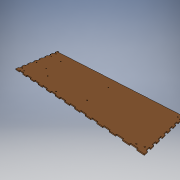
# Autodesk Inventor part: tavolaBase
Saved by Autodesk Inventor 2018.3 (Build 223284000, 284)
## iProperties
Created: 2019-03-04
Part Number: tavolaBase
Material: Generico
Document SubType Name: Modeling
Designer: AlfyPc
Density: 1 g/cm^3
Appearance: Frassino bianco - Giava
Author: AlfyPc
Autodesk Inventor part; units mm, degrees
ref_plane "YZ Plane" through (0, 0, 0) normal (1, 0, 0) x (0, 1, 0)
ref_plane "XZ Plane" through (0, 0, 0) normal (0, 1, 0) x (-1, 0, 0)
ref_plane "XY Plane" through (0, 0, 0) normal (0, 0, 1) x (1, 0, 0)
sketch "Schizzo1" plane through (0, 0, 0) normal (0, 0, 1) x (1, 0, 0)
  line L0 (233.5, -78.5) -> (-233.5, -78.5)
  line L1 (-233.5, -78.5) -> (-233.5, 78.5)
  line L2 (-233.5, 78.5) -> (233.5, 78.5)
  line L3 (233.5, 78.5) -> (233.5, -78.5)
  line L4 (233.5, -78.5) -> (-233.5, 78.5) construction
  line L5 (-233.5, -78.5) -> (233.5, 78.5) construction
  point P0 (0, 0)
  dimension "d0" = 467
  dimension "d1" = 157
  constraints: 12 end point, 2 midpoint, 2 parallel, 1 horizontal, 1 perpendicular
  measures "d0" distance of L0.start L0.end
  measures "d1" distance of L0.end L1.end
extrude "Estrusione1" add sketch "Schizzo1" against normal blind 4
sketch "Schizzo3" plane through (0, 0, 0) normal (0, 0, 1) x (1, 0, 0)
  line L0 (233.5, -78.5) -> (-233.5, -78.5) projected
  line L1 (233.5, 78.5) -> (233.5, -78.5) projected
  line L2 (-233.5, 78.5) -> (233.5, 78.5) projected
  line L3 (-233.5, -78.5) -> (-233.5, 78.5) projected
  line L4 (-237.5, -82.5) -> (237.5, -82.5) construction
  line L5 (237.5, -82.5) -> (237.5, 82.5) construction
  line L6 (237.5, 82.5) -> (-237.5, 82.5) construction
  line L7 (-237.5, 82.5) -> (-237.5, -82.5) construction
  line L8 (237.5, -82.5) -> (218.5, -82.5)
  line L9 (218.5, -82.5) -> (218.5, -78.5)
  line L10 (218.5, -78.5) -> (237.5, -78.5)
  line L11 (237.5, -78.5) -> (237.5, -82.5)
  line L12 (237.5, 82.5) -> (218.5, 82.5)
  line L13 (218.5, 82.5) -> (218.5, 78.5)
  line L14 (218.5, 78.5) -> (237.5, 78.5)
  line L15 (237.5, 78.5) -> (237.5, 82.5)
  line L16 (237.5, -82.5) -> (233.5, -82.5)
  line L17 (233.5, -82.5) -> (233.5, -71.5)
  line L18 (233.5, -71.5) -> (237.5, -71.5)
  line L19 (237.5, -71.5) -> (237.5, -82.5)
  line L20 (-237.5, -82.5) -> (-233.5, -82.5)
  line L21 (-233.5, -82.5) -> (-233.5, -71.5)
  line L22 (-233.5, -71.5) -> (-237.5, -71.5)
  line L23 (-237.5, -71.5) -> (-237.5, -82.5)
  line L24 (218.5, -78.5) -> (218.5, -82.5)
  line L25 (218.5, -82.5) -> (214.5, -82.5)
  line L26 (199.5, -82.5) -> (199.5, -78.5)
  line L27 (199.5, -78.5) -> (218.5, -78.5)
  line L28 (218.5, -82.5) -> (199.5, -82.5)
  line L29 (199.5, 82.5) -> (199.5, 78.5)
  line L30 (199.5, 78.5) -> (218.5, 78.5)
  line L31 (218.5, 78.5) -> (218.5, 82.5)
  line L32 (218.5, 82.5) -> (199.5, 82.5)
  line L33 (199.5, -78.5) -> (199.5, -82.5)
  line L34 (199.5, -82.5) -> (195.5, -82.5)
  line L35 (180.5, -82.5) -> (180.5, -78.5)
  line L36 (180.5, -78.5) -> (199.5, -78.5)
  line L37 (199.5, -82.5) -> (180.5, -82.5)
  line L38 (180.5, 82.5) -> (180.5, 78.5)
  line L39 (180.5, 78.5) -> (199.5, 78.5)
  line L40 (199.5, 78.5) -> (199.5, 82.5)
  line L41 (199.5, 82.5) -> (180.5, 82.5)
  line L42 (180.5, -78.5) -> (180.5, -82.5)
  line L43 (180.5, -82.5) -> (176.5, -82.5)
  line L44 (161.5, -82.5) -> (161.5, -78.5)
  line L45 (161.5, -78.5) -> (180.5, -78.5)
  line L46 (180.5, -82.5) -> (161.5, -82.5)
  line L47 (161.5, 82.5) -> (161.5, 78.5)
  line L48 (161.5, 78.5) -> (180.5, 78.5)
  line L49 (180.5, 78.5) -> (180.5, 82.5)
  line L50 (180.5, 82.5) -> (161.5, 82.5)
  line L51 (161.5, -78.5) -> (161.5, -82.5)
  line L52 (161.5, -82.5) -> (157.5, -82.5)
  line L53 (142.5, -82.5) -> (142.5, -78.5)
  line L54 (142.5, -78.5) -> (161.5, -78.5)
  line L55 (161.5, -82.5) -> (142.5, -82.5)
  line L56 (142.5, 82.5) -> (142.5, 78.5)
  line L57 (142.5, 78.5) -> (161.5, 78.5)
  line L58 (161.5, 78.5) -> (161.5, 82.5)
  line L59 (161.5, 82.5) -> (142.5, 82.5)
  line L60 (142.5, -78.5) -> (142.5, -82.5)
  line L61 (142.5, -82.5) -> (138.5, -82.5)
  line L62 (123.5, -82.5) -> (123.5, -78.5)
  line L63 (123.5, -78.5) -> (142.5, -78.5)
  line L64 (142.5, -82.5) -> (123.5, -82.5)
  line L65 (123.5, 82.5) -> (123.5, 78.5)
  line L66 (123.5, 78.5) -> (142.5, 78.5)
  line L67 (142.5, 78.5) -> (142.5, 82.5)
  line L68 (142.5, 82.5) -> (123.5, 82.5)
  line L69 (123.5, -78.5) -> (123.5, -82.5)
  line L70 (123.5, -82.5) -> (119.5, -82.5)
  line L71 (104.5, -82.5) -> (104.5, -78.5)
  line L72 (104.5, -78.5) -> (123.5, -78.5)
  line L73 (123.5, -82.5) -> (104.5, -82.5)
  line L74 (104.5, 82.5) -> (104.5, 78.5)
  line L75 (104.5, 78.5) -> (123.5, 78.5)
  line L76 (123.5, 78.5) -> (123.5, 82.5)
  line L77 (123.5, 82.5) -> (104.5, 82.5)
  line L78 (104.5, -78.5) -> (104.5, -82.5)
  line L79 (104.5, -82.5) -> (100.5, -82.5)
  line L80 (85.5, -82.5) -> (85.5, -78.5)
  line L81 (85.5, -78.5) -> (104.5, -78.5)
  line L82 (104.5, -82.5) -> (85.5, -82.5)
  line L83 (85.5, 82.5) -> (85.5, 78.5)
  line L84 (85.5, 78.5) -> (104.5, 78.5)
  line L85 (104.5, 78.5) -> (104.5, 82.5)
  line L86 (104.5, 82.5) -> (85.5, 82.5)
  line L87 (85.5, -78.5) -> (85.5, -82.5)
  line L88 (85.5, -82.5) -> (81.5, -82.5)
  line L89 (66.5, -82.5) -> (66.5, -78.5)
  line L90 (66.5, -78.5) -> (85.5, -78.5)
  line L91 (85.5, -82.5) -> (66.5, -82.5)
  line L92 (66.5, 82.5) -> (66.5, 78.5)
  line L93 (66.5, 78.5) -> (85.5, 78.5)
  line L94 (85.5, 78.5) -> (85.5, 82.5)
  line L95 (85.5, 82.5) -> (66.5, 82.5)
  line L96 (66.5, -78.5) -> (66.5, -82.5)
  line L97 (66.5, -82.5) -> (62.5, -82.5)
  line L98 (47.5, -82.5) -> (47.5, -78.5)
  line L99 (47.5, -78.5) -> (66.5, -78.5)
  line L100 (66.5, -82.5) -> (47.5, -82.5)
  line L101 (47.5, 82.5) -> (47.5, 78.5)
  line L102 (47.5, 78.5) -> (66.5, 78.5)
  line L103 (66.5, 78.5) -> (66.5, 82.5)
  line L104 (66.5, 82.5) -> (47.5, 82.5)
  line L105 (47.5, -78.5) -> (47.5, -82.5)
  line L106 (47.5, -82.5) -> (43.5, -82.5)
  line L107 (28.5, -82.5) -> (28.5, -78.5)
  line L108 (28.5, -78.5) -> (47.5, -78.5)
  line L109 (47.5, -82.5) -> (28.5, -82.5)
  line L110 (28.5, 82.5) -> (28.5, 78.5)
  line L111 (28.5, 78.5) -> (47.5, 78.5)
  line L112 (47.5, 78.5) -> (47.5, 82.5)
  line L113 (47.5, 82.5) -> (28.5, 82.5)
  line L114 (28.5, -78.5) -> (28.5, -82.5)
  line L115 (28.5, -82.5) -> (24.5, -82.5)
  line L116 (9.5, -82.5) -> (9.5, -78.5)
  line L117 (9.5, -78.5) -> (28.5, -78.5)
  line L118 (28.5, -82.5) -> (9.5, -82.5)
  line L119 (9.5, 82.5) -> (9.5, 78.5)
  line L120 (9.5, 78.5) -> (28.5, 78.5)
  line L121 (28.5, 78.5) -> (28.5, 82.5)
  line L122 (28.5, 82.5) -> (9.5, 82.5)
  line L123 (9.5, -78.5) -> (9.5, -82.5)
  line L124 (9.5, -82.5) -> (5.5, -82.5)
  line L125 (-9.5, -82.5) -> (-9.5, -78.5)
  line L126 (-9.5, -78.5) -> (9.5, -78.5)
  line L127 (9.5, -82.5) -> (-9.5, -82.5)
  line L128 (-9.5, 82.5) -> (-9.5, 78.5)
  line L129 (-9.5, 78.5) -> (9.5, 78.5)
  line L130 (9.5, 78.5) -> (9.5, 82.5)
  line L131 (9.5, 82.5) -> (-9.5, 82.5)
  line L132 (-9.5, -78.5) -> (-9.5, -82.5)
  line L133 (-9.5, -82.5) -> (-13.5, -82.5)
  line L134 (-28.5, -82.5) -> (-28.5, -78.5)
  line L135 (-28.5, -78.5) -> (-9.5, -78.5)
  line L136 (-9.5, -82.5) -> (-28.5, -82.5)
  line L137 (-28.5, 82.5) -> (-28.5, 78.5)
  line L138 (-28.5, 78.5) -> (-9.5, 78.5)
  line L139 (-9.5, 78.5) -> (-9.5, 82.5)
  line L140 (-9.5, 82.5) -> (-28.5, 82.5)
  line L141 (-28.5, -78.5) -> (-28.5, -82.5)
  line L142 (-28.5, -82.5) -> (-32.5, -82.5)
  line L143 (-47.5, -82.5) -> (-47.5, -78.5)
  line L144 (-47.5, -78.5) -> (-28.5, -78.5)
  line L145 (-28.5, -82.5) -> (-47.5, -82.5)
  line L146 (-47.5, 82.5) -> (-47.5, 78.5)
  line L147 (-47.5, 78.5) -> (-28.5, 78.5)
  line L148 (-28.5, 78.5) -> (-28.5, 82.5)
  line L149 (-28.5, 82.5) -> (-47.5, 82.5)
  line L150 (-47.5, -78.5) -> (-47.5, -82.5)
  line L151 (-47.5, -82.5) -> (-51.5, -82.5)
  line L152 (-66.5, -82.5) -> (-66.5, -78.5)
  line L153 (-66.5, -78.5) -> (-47.5, -78.5)
  line L154 (-47.5, -82.5) -> (-66.5, -82.5)
  line L155 (-66.5, 82.5) -> (-66.5, 78.5)
  line L156 (-66.5, 78.5) -> (-47.5, 78.5)
  line L157 (-47.5, 78.5) -> (-47.5, 82.5)
  line L158 (-47.5, 82.5) -> (-66.5, 82.5)
  line L159 (-66.5, -78.5) -> (-66.5, -82.5)
  line L160 (-66.5, -82.5) -> (-70.5, -82.5)
  line L161 (-85.5, -82.5) -> (-85.5, -78.5)
  line L162 (-85.5, -78.5) -> (-66.5, -78.5)
  line L163 (-66.5, -82.5) -> (-85.5, -82.5)
  line L164 (-85.5, 82.5) -> (-85.5, 78.5)
  line L165 (-85.5, 78.5) -> (-66.5, 78.5)
  line L166 (-66.5, 78.5) -> (-66.5, 82.5)
  line L167 (-66.5, 82.5) -> (-85.5, 82.5)
  line L168 (-85.5, -78.5) -> (-85.5, -82.5)
  line L169 (-85.5, -82.5) -> (-89.5, -82.5)
  line L170 (-104.5, -82.5) -> (-104.5, -78.5)
  line L171 (-104.5, -78.5) -> (-85.5, -78.5)
  line L172 (-85.5, -82.5) -> (-104.5, -82.5)
  line L173 (-104.5, 82.5) -> (-104.5, 78.5)
  line L174 (-104.5, 78.5) -> (-85.5, 78.5)
  line L175 (-85.5, 78.5) -> (-85.5, 82.5)
  line L176 (-85.5, 82.5) -> (-104.5, 82.5)
  line L177 (-104.5, -78.5) -> (-104.5, -82.5)
  line L178 (-104.5, -82.5) -> (-108.5, -82.5)
  line L179 (-123.5, -82.5) -> (-123.5, -78.5)
  line L180 (-123.5, -78.5) -> (-104.5, -78.5)
  line L181 (-104.5, -82.5) -> (-123.5, -82.5)
  line L182 (-123.5, 82.5) -> (-123.5, 78.5)
  line L183 (-123.5, 78.5) -> (-104.5, 78.5)
  line L184 (-104.5, 78.5) -> (-104.5, 82.5)
  line L185 (-104.5, 82.5) -> (-123.5, 82.5)
  line L186 (-123.5, -78.5) -> (-123.5, -82.5)
  line L187 (-123.5, -82.5) -> (-127.5, -82.5)
  line L188 (-142.5, -82.5) -> (-142.5, -78.5)
  line L189 (-142.5, -78.5) -> (-123.5, -78.5)
  line L190 (-123.5, -82.5) -> (-142.5, -82.5)
  line L191 (-142.5, 82.5) -> (-142.5, 78.5)
  line L192 (-142.5, 78.5) -> (-123.5, 78.5)
  line L193 (-123.5, 78.5) -> (-123.5, 82.5)
  line L194 (-123.5, 82.5) -> (-142.5, 82.5)
  line L195 (-142.5, -78.5) -> (-142.5, -82.5)
  line L196 (-142.5, -82.5) -> (-146.5, -82.5)
  line L197 (-161.5, -82.5) -> (-161.5, -78.5)
  line L198 (-161.5, -78.5) -> (-142.5, -78.5)
  line L199 (-142.5, -82.5) -> (-161.5, -82.5)
  line L200 (-161.5, 82.5) -> (-161.5, 78.5)
  line L201 (-161.5, 78.5) -> (-142.5, 78.5)
  line L202 (-142.5, 78.5) -> (-142.5, 82.5)
  line L203 (-142.5, 82.5) -> (-161.5, 82.5)
  line L204 (-161.5, -78.5) -> (-161.5, -82.5)
  line L205 (-161.5, -82.5) -> (-165.5, -82.5)
  line L206 (-180.5, -82.5) -> (-180.5, -78.5)
  line L207 (-180.5, -78.5) -> (-161.5, -78.5)
  line L208 (-161.5, -82.5) -> (-180.5, -82.5)
  line L209 (-180.5, 82.5) -> (-180.5, 78.5)
  line L210 (-180.5, 78.5) -> (-161.5, 78.5)
  line L211 (-161.5, 78.5) -> (-161.5, 82.5)
  line L212 (-161.5, 82.5) -> (-180.5, 82.5)
  line L213 (-180.5, -78.5) -> (-180.5, -82.5)
  line L214 (-180.5, -82.5) -> (-184.5, -82.5)
  line L215 (-199.5, -82.5) -> (-199.5, -78.5)
  line L216 (-199.5, -78.5) -> (-180.5, -78.5)
  line L217 (-180.5, -82.5) -> (-199.5, -82.5)
  line L218 (-199.5, 82.5) -> (-199.5, 78.5)
  line L219 (-199.5, 78.5) -> (-180.5, 78.5)
  line L220 (-180.5, 78.5) -> (-180.5, 82.5)
  line L221 (-180.5, 82.5) -> (-199.5, 82.5)
  line L222 (-199.5, -78.5) -> (-199.5, -82.5)
  line L223 (-199.5, -82.5) -> (-203.5, -82.5)
  line L224 (-218.5, -82.5) -> (-218.5, -78.5)
  line L225 (-218.5, -78.5) -> (-199.5, -78.5)
  line L226 (-199.5, -82.5) -> (-218.5, -82.5)
  line L227 (-218.5, 82.5) -> (-218.5, 78.5)
  line L228 (-218.5, 78.5) -> (-199.5, 78.5)
  line L229 (-199.5, 78.5) -> (-199.5, 82.5)
  line L230 (-199.5, 82.5) -> (-218.5, 82.5)
  line L231 (-218.5, -78.5) -> (-218.5, -82.5)
  line L232 (-218.5, -82.5) -> (-222.5, -82.5)
  line L233 (-237.5, -82.5) -> (-237.5, -78.5)
  line L234 (-237.5, -78.5) -> (-218.5, -78.5)
  line L235 (-218.5, -82.5) -> (-237.5, -82.5)
  line L236 (-237.5, 82.5) -> (-237.5, 78.5)
  line L237 (-237.5, 78.5) -> (-218.5, 78.5)
  line L238 (-218.5, 78.5) -> (-218.5, 82.5)
  line L239 (-218.5, 82.5) -> (-237.5, 82.5)
  line L240 (237.5, -67.5) -> (237.5, -71.5)
  line L241 (237.5, -71.5) -> (233.5, -71.5)
  line L242 (233.5, -60.5) -> (237.5, -60.5)
  line L243 (237.5, -60.5) -> (237.5, -71.5)
  line L244 (233.5, -71.5) -> (233.5, -60.5)
  line L245 (-237.5, -71.5) -> (-233.5, -71.5)
  line L246 (-233.5, -71.5) -> (-233.5, -60.5)
  line L247 (-233.5, -60.5) -> (-237.5, -60.5)
  line L248 (-237.5, -60.5) -> (-237.5, -71.5)
  line L249 (-237.5, -71.5) -> (-237.5, -67.5)
  line L250 (237.5, -56.5) -> (237.5, -60.5)
  line L251 (237.5, -60.5) -> (233.5, -60.5)
  line L252 (233.5, -49.5) -> (237.5, -49.5)
  line L253 (237.5, -49.5) -> (237.5, -60.5)
  line L254 (233.5, -60.5) -> (233.5, -49.5)
  line L255 (-237.5, -60.5) -> (-233.5, -60.5)
  line L256 (-233.5, -60.5) -> (-233.5, -49.5)
  line L257 (-233.5, -49.5) -> (-237.5, -49.5)
  line L258 (-237.5, -49.5) -> (-237.5, -60.5)
  line L259 (-237.5, -60.5) -> (-237.5, -56.5)
  line L260 (237.5, -45.5) -> (237.5, -49.5)
  line L261 (237.5, -49.5) -> (233.5, -49.5)
  line L262 (233.5, -38.5) -> (237.5, -38.5)
  line L263 (237.5, -38.5) -> (237.5, -49.5)
  line L264 (233.5, -49.5) -> (233.5, -38.5)
  line L265 (-237.5, -49.5) -> (-233.5, -49.5)
  line L266 (-233.5, -49.5) -> (-233.5, -38.5)
  line L267 (-233.5, -38.5) -> (-237.5, -38.5)
  line L268 (-237.5, -38.5) -> (-237.5, -49.5)
  line L269 (-237.5, -49.5) -> (-237.5, -45.5)
  line L270 (237.5, -34.5) -> (237.5, -38.5)
  line L271 (237.5, -38.5) -> (233.5, -38.5)
  line L272 (233.5, -27.5) -> (237.5, -27.5)
  line L273 (237.5, -27.5) -> (237.5, -38.5)
  line L274 (233.5, -38.5) -> (233.5, -27.5)
  line L275 (-237.5, -38.5) -> (-233.5, -38.5)
  line L276 (-233.5, -38.5) -> (-233.5, -27.5)
  line L277 (-233.5, -27.5) -> (-237.5, -27.5)
  line L278 (-237.5, -27.5) -> (-237.5, -38.5)
  line L279 (-237.5, -38.5) -> (-237.5, -34.5)
  line L280 (237.5, -23.5) -> (237.5, -27.5)
  line L281 (237.5, -27.5) -> (233.5, -27.5)
  line L282 (233.5, -16.5) -> (237.5, -16.5)
  line L283 (237.5, -16.5) -> (237.5, -27.5)
  line L284 (233.5, -27.5) -> (233.5, -16.5)
  line L285 (-237.5, -27.5) -> (-233.5, -27.5)
  line L286 (-233.5, -27.5) -> (-233.5, -16.5)
  line L287 (-233.5, -16.5) -> (-237.5, -16.5)
  line L288 (-237.5, -16.5) -> (-237.5, -27.5)
  line L289 (-237.5, -27.5) -> (-237.5, -23.5)
  line L290 (237.5, -12.5) -> (237.5, -16.5)
  line L291 (237.5, -16.5) -> (233.5, -16.5)
  line L292 (233.5, -5.5) -> (237.5, -5.5)
  line L293 (237.5, -5.5) -> (237.5, -16.5)
  line L294 (233.5, -16.5) -> (233.5, -5.5)
  line L295 (-237.5, -16.5) -> (-233.5, -16.5)
  line L296 (-233.5, -16.5) -> (-233.5, -5.5)
  line L297 (-233.5, -5.5) -> (-237.5, -5.5)
  line L298 (-237.5, -5.5) -> (-237.5, -16.5)
  line L299 (-237.5, -16.5) -> (-237.5, -12.5)
  line L300 (237.5, -1.5) -> (237.5, -5.5)
  line L301 (237.5, -5.5) -> (233.5, -5.5)
  line L302 (233.5, 5.5) -> (237.5, 5.5)
  line L303 (237.5, 5.5) -> (237.5, -5.5)
  line L304 (233.5, -5.5) -> (233.5, 5.5)
  line L305 (-237.5, -5.5) -> (-233.5, -5.5)
  line L306 (-233.5, -5.5) -> (-233.5, 5.5)
  line L307 (-233.5, 5.5) -> (-237.5, 5.5)
  line L308 (-237.5, 5.5) -> (-237.5, -5.5)
  line L309 (-237.5, -5.5) -> (-237.5, -1.5)
  line L310 (237.5, 9.5) -> (237.5, 5.5)
  line L311 (237.5, 5.5) -> (233.5, 5.5)
  line L312 (233.5, 16.5) -> (237.5, 16.5)
  line L313 (237.5, 16.5) -> (237.5, 5.5)
  line L314 (233.5, 5.5) -> (233.5, 16.5)
  line L315 (-237.5, 5.5) -> (-233.5, 5.5)
  line L316 (-233.5, 5.5) -> (-233.5, 16.5)
  line L317 (-233.5, 16.5) -> (-237.5, 16.5)
  line L318 (-237.5, 16.5) -> (-237.5, 5.5)
  line L319 (-237.5, 5.5) -> (-237.5, 9.5)
  line L320 (237.5, 20.5) -> (237.5, 16.5)
  line L321 (237.5, 16.5) -> (233.5, 16.5)
  line L322 (233.5, 27.5) -> (237.5, 27.5)
  line L323 (237.5, 27.5) -> (237.5, 16.5)
  line L324 (233.5, 16.5) -> (233.5, 27.5)
  line L325 (-237.5, 16.5) -> (-233.5, 16.5)
  line L326 (-233.5, 16.5) -> (-233.5, 27.5)
  line L327 (-233.5, 27.5) -> (-237.5, 27.5)
  line L328 (-237.5, 27.5) -> (-237.5, 16.5)
  line L329 (-237.5, 16.5) -> (-237.5, 20.5)
  line L330 (237.5, 31.5) -> (237.5, 27.5)
  line L331 (237.5, 27.5) -> (233.5, 27.5)
  line L332 (233.5, 38.5) -> (237.5, 38.5)
  line L333 (237.5, 38.5) -> (237.5, 27.5)
  line L334 (233.5, 27.5) -> (233.5, 38.5)
  line L335 (-237.5, 27.5) -> (-233.5, 27.5)
  line L336 (-233.5, 27.5) -> (-233.5, 38.5)
  line L337 (-233.5, 38.5) -> (-237.5, 38.5)
  line L338 (-237.5, 38.5) -> (-237.5, 27.5)
  line L339 (-237.5, 27.5) -> (-237.5, 31.5)
  line L340 (237.5, 42.5) -> (237.5, 38.5)
  line L341 (237.5, 38.5) -> (233.5, 38.5)
  line L342 (233.5, 49.5) -> (237.5, 49.5)
  line L343 (237.5, 49.5) -> (237.5, 38.5)
  line L344 (233.5, 38.5) -> (233.5, 49.5)
  line L345 (-237.5, 38.5) -> (-233.5, 38.5)
  line L346 (-233.5, 38.5) -> (-233.5, 49.5)
  line L347 (-233.5, 49.5) -> (-237.5, 49.5)
  line L348 (-237.5, 49.5) -> (-237.5, 38.5)
  line L349 (-237.5, 38.5) -> (-237.5, 42.5)
  line L350 (237.5, 53.5) -> (237.5, 49.5)
  line L351 (237.5, 49.5) -> (233.5, 49.5)
  line L352 (233.5, 60.5) -> (237.5, 60.5)
  line L353 (237.5, 60.5) -> (237.5, 49.5)
  line L354 (233.5, 49.5) -> (233.5, 60.5)
  line L355 (-237.5, 49.5) -> (-233.5, 49.5)
  line L356 (-233.5, 49.5) -> (-233.5, 60.5)
  line L357 (-233.5, 60.5) -> (-237.5, 60.5)
  line L358 (-237.5, 60.5) -> (-237.5, 49.5)
  line L359 (-237.5, 49.5) -> (-237.5, 53.5)
  line L360 (237.5, 64.5) -> (237.5, 60.5)
  line L361 (237.5, 60.5) -> (233.5, 60.5)
  line L362 (233.5, 71.5) -> (237.5, 71.5)
  line L363 (237.5, 71.5) -> (237.5, 60.5)
  line L364 (233.5, 60.5) -> (233.5, 71.5)
  line L365 (-237.5, 60.5) -> (-233.5, 60.5)
  line L366 (-233.5, 60.5) -> (-233.5, 71.5)
  line L367 (-233.5, 71.5) -> (-237.5, 71.5)
  line L368 (-237.5, 71.5) -> (-237.5, 60.5)
  line L369 (-237.5, 60.5) -> (-237.5, 64.5)
  line L370 (237.5, 75.5) -> (237.5, 71.5)
  line L371 (237.5, 71.5) -> (233.5, 71.5)
  line L372 (233.5, 82.5) -> (237.5, 82.5)
  line L373 (237.5, 82.5) -> (237.5, 71.5)
  line L374 (233.5, 71.5) -> (233.5, 82.5)
  line L375 (-237.5, 71.5) -> (-233.5, 71.5)
  line L376 (-233.5, 71.5) -> (-233.5, 82.5)
  line L377 (-233.5, 82.5) -> (-237.5, 82.5)
  line L378 (-237.5, 82.5) -> (-237.5, 71.5)
  line L379 (-237.5, 71.5) -> (-237.5, 75.5)
  point P0 (0, 0)
  point P1 (214.5, -78.5)
  point P2 (214.5, 78.5)
  point P3 (195.5, -78.5)
  point P4 (195.5, 78.5)
  point P5 (176.5, -78.5)
  point P6 (176.5, 78.5)
  point P7 (157.5, -78.5)
  point P8 (157.5, 78.5)
  point P9 (138.5, -78.5)
  point P10 (138.5, 78.5)
  point P11 (119.5, -78.5)
  point P12 (119.5, 78.5)
  point P13 (100.5, -78.5)
  point P14 (100.5, 78.5)
  point P15 (81.5, -78.5)
  point P16 (81.5, 78.5)
  point P17 (62.5, -78.5)
  point P18 (62.5, 78.5)
  point P19 (43.5, -78.5)
  point P20 (43.5, 78.5)
  point P21 (24.5, -78.5)
  point P22 (24.5, 78.5)
  point P23 (5.5, -78.5)
  point P24 (5.5, 78.5)
  point P25 (-13.5, -78.5)
  point P26 (-13.5, 78.5)
  point P27 (-32.5, -78.5)
  point P28 (-32.5, 78.5)
  point P29 (-51.5, -78.5)
  point P30 (-51.5, 78.5)
  point P31 (-70.5, -78.5)
  point P32 (-70.5, 78.5)
  point P33 (-89.5, -78.5)
  point P34 (-89.5, 78.5)
  point P35 (-108.5, -78.5)
  point P36 (-108.5, 78.5)
  point P37 (-127.5, -78.5)
  point P38 (-127.5, 78.5)
  point P39 (-146.5, -78.5)
  point P40 (-146.5, 78.5)
  point P41 (-165.5, -78.5)
  point P42 (-165.5, 78.5)
  point P43 (-184.5, -78.5)
  point P44 (-184.5, 78.5)
  point P45 (-203.5, -78.5)
  point P46 (-203.5, 78.5)
  point P47 (-222.5, -78.5)
  point P48 (-222.5, 78.5)
  point P49 (233.5, -67.5)
  point P50 (-233.5, -67.5)
  point P51 (233.5, -56.5)
  point P52 (-233.5, -56.5)
  point P53 (233.5, -45.5)
  point P54 (-233.5, -45.5)
  point P55 (233.5, -34.5)
  point P56 (-233.5, -34.5)
  point P57 (233.5, -23.5)
  point P58 (-233.5, -23.5)
  point P59 (233.5, -12.5)
  point P60 (-233.5, -12.5)
  point P61 (233.5, -1.5)
  point P62 (-233.5, -1.5)
  point P63 (233.5, 9.5)
  point P64 (-233.5, 9.5)
  point P65 (233.5, 20.5)
  point P66 (-233.5, 20.5)
  point P67 (233.5, 31.5)
  point P68 (-233.5, 31.5)
  point P69 (233.5, 42.5)
  point P70 (-233.5, 42.5)
  point P71 (233.5, 53.5)
  point P72 (-233.5, 53.5)
  point P73 (233.5, 64.5)
  point P74 (-233.5, 64.5)
  point P75 (233.5, 75.5)
  point P76 (-233.5, 75.5)
  dimension "d28" = 4
  dimension "d29" = 475
  dimension "d30" = 165
  dimension "d31" = 19
  dimension "d32" = 4
  dimension "d33" = 19
  dimension "d34" = 4
  dimension "d35" = 4
  dimension "d36" = 11
  dimension "d37" = 4
  dimension "d38" = 11
  dimension "d41" = 19
  dimension "d48" = 11
  constraints: 752 end point, 8 parallel, 5 horizontal, 4 perpendicular, 1 vertical, 805 other
  measures "d28" distance between parallel lines of L0 L4
  measures "d29" distance of L4.start L4.end
  measures "d30" distance of L4.end L5.end
  measures "d31" distance of L9.end L10.end
  measures "d32" distance of L8.end L9.end
  measures "d33" distance of L14.end L13.end
  measures "d34" distance of L13.end L12.end
  measures "d35" distance of L17.end L18.end
  measures "d36" distance of L16.end L17.end
  measures "d37" distance of L22.end L21.end
  measures "d38" distance of L21.end L20.end
  measures "d41" distance of L10.end L24.start
  measures "d48" distance of L0.start point (233.5, -67.5)
extrude "Estrusione2" add sketch "Schizzo3" against normal up to surface (4 mm away) contours L17 L8 L9 L0 | L1 L18 L19 L10 | L10 L11 L8 L17 | L26 L34 L37 L35 L0 | L1 L252 L253 L250 L242 | L44 L52 L55 L53 L0 | L1 L272 L273 L270 L262 | L62 L70 L73 L71 L0 | L1 L292 L293 L290 L282 | L80 L88 L91 L89 L0 | L1 L312 L313 L310 L302 | L98 L106 L109 L107 L0 | L1 L332 L333 L330 L322 | L116 L124 L127 L125 L0 | L1 L352 L353 L350 L342 | L134 L142 L145 L143 L0 | L1 L14 L373 L370 L362 | L374 L12 L15 L14 | L152 L160 L163 L161 L0 | L170 L178 L181 L179 L0 | L188 L196 L199 L197 L0 | L206 L214 L217 L215 L0 | L224 L232 L235 L21 L0 | L234 L23 L22 L3 | L21 L20 L23 L234 | L247 L258 L257 L3 | L267 L278 L277 L3 | L287 L298 L297 L3 | L307 L318 L317 L3 | L327 L338 L337 L3 | L347 L358 L357 L3 | L367 L378 L237 L3 | L237 L236 L239 L376
sketch "Schizzo4" plane through (0, 0, 0) normal (0, 0, 1) x (1, 0, 0)
  circle A0 centre (29.075, -39.395) radius 1.5
  circle A1 centre (29.075, 41.885) radius 1.5
  circle A2 centre (-135.39, -38.76) radius 1.5
  circle A3 centre (-173.97, 42.5) radius 1.375
  circle A4 centre (-222.97, 42.5) radius 1.375
  circle A5 centre (-173.97, -15.5) radius 1.375
  circle A6 centre (-222.97, -15.5) radius 1.375
  point P0 (0, 0)
extrude "Estrusione3" cut sketch "Schizzo4" against normal blind 10
sketch "Schizzo5" plane through (0, 0, 0) normal (0, 0, 1) x (1, 0, 0)
  circle A0 centre (29.075, 41.885) radius 1.5 projected
  circle A1 centre (-222.97, -15.5) radius 1.375 projected
  circle A2 centre (-222.97, 42.5) radius 1.375 projected
  circle A3 centre (-173.97, 42.5) radius 1.375 projected
  circle A4 centre (-173.97, -15.5) radius 1.375 projected
  circle A5 centre (29.075, -39.395) radius 1.5 projected
  circle A6 centre (-135.39, -38.76) radius 1.5 projected
  line L0 (218.5, -82.5) -> (218.5, -78.5) projected
  line L1 (237.5, -82.5) -> (218.5, -82.5) projected
  line L2 (237.5, -71.5) -> (237.5, -82.5) projected
  line L3 (233.5, -71.5) -> (237.5, -71.5) projected
  line L4 (233.5, -60.5) -> (233.5, -71.5) projected
  line L5 (237.5, -60.5) -> (233.5, -60.5) projected
  line L6 (237.5, -49.5) -> (237.5, -60.5) projected
  line L7 (233.5, -49.5) -> (237.5, -49.5) projected
  line L8 (233.5, -38.5) -> (233.5, -49.5) projected
  line L9 (237.5, -38.5) -> (233.5, -38.5) projected
  line L10 (237.5, -27.5) -> (237.5, -38.5) projected
  line L11 (233.5, -27.5) -> (237.5, -27.5) projected
  line L12 (233.5, -16.5) -> (233.5, -27.5) projected
  line L13 (237.5, -16.5) -> (233.5, -16.5) projected
  line L14 (237.5, -5.5) -> (237.5, -16.5) projected
  line L15 (233.5, -5.5) -> (237.5, -5.5) projected
  line L16 (233.5, 5.5) -> (233.5, -5.5) projected
  line L17 (237.5, 5.5) -> (233.5, 5.5) projected
  line L18 (237.5, 16.5) -> (237.5, 5.5) projected
  line L19 (233.5, 16.5) -> (237.5, 16.5) projected
  line L20 (233.5, 27.5) -> (233.5, 16.5) projected
  line L21 (237.5, 27.5) -> (233.5, 27.5) projected
  line L22 (237.5, 38.5) -> (237.5, 27.5) projected
  line L23 (233.5, 38.5) -> (237.5, 38.5) projected
  line L24 (233.5, 49.5) -> (233.5, 38.5) projected
  line L25 (237.5, 49.5) -> (233.5, 49.5) projected
  line L26 (237.5, 60.5) -> (237.5, 49.5) projected
  line L27 (233.5, 60.5) -> (237.5, 60.5) projected
  line L28 (233.5, 71.5) -> (233.5, 60.5) projected
  line L29 (237.5, 71.5) -> (233.5, 71.5) projected
  line L30 (237.5, 82.5) -> (237.5, 71.5) projected
  line L31 (233.5, 82.5) -> (237.5, 82.5) projected
  line L32 (233.5, 78.5) -> (233.5, 82.5) projected
  line L33 (-233.5, 78.5) -> (233.5, 78.5) projected
  line L34 (-233.5, 78.5) -> (-233.5, 82.5) projected
  line L35 (-233.5, 82.5) -> (-237.5, 82.5) projected
  line L36 (-237.5, 82.5) -> (-237.5, 71.5) projected
  line L37 (-237.5, 71.5) -> (-233.5, 71.5) projected
  line L38 (-233.5, 60.5) -> (-233.5, 71.5) projected
  line L39 (-233.5, 60.5) -> (-237.5, 60.5) projected
  line L40 (-237.5, 60.5) -> (-237.5, 49.5) projected
  line L41 (-237.5, 49.5) -> (-233.5, 49.5) projected
  line L42 (-233.5, 38.5) -> (-233.5, 49.5) projected
  line L43 (-233.5, 38.5) -> (-237.5, 38.5) projected
  line L44 (-237.5, 38.5) -> (-237.5, 27.5) projected
  line L45 (-237.5, 27.5) -> (-233.5, 27.5) projected
  line L46 (-233.5, 16.5) -> (-233.5, 27.5) projected
  line L47 (-233.5, 16.5) -> (-237.5, 16.5) projected
  line L48 (-237.5, 16.5) -> (-237.5, 5.5) projected
  line L49 (-237.5, 5.5) -> (-233.5, 5.5) projected
  line L50 (-233.5, -5.5) -> (-233.5, 5.5) projected
  line L51 (-233.5, -5.5) -> (-237.5, -5.5) projected
  line L52 (-237.5, -5.5) -> (-237.5, -16.5) projected
  line L53 (-237.5, -16.5) -> (-233.5, -16.5) projected
  line L54 (-233.5, -27.5) -> (-233.5, -16.5) projected
  line L55 (-233.5, -27.5) -> (-237.5, -27.5) projected
  line L56 (-237.5, -27.5) -> (-237.5, -38.5) projected
  line L57 (-237.5, -38.5) -> (-233.5, -38.5) projected
  line L58 (-233.5, -49.5) -> (-233.5, -38.5) projected
  line L59 (-233.5, -49.5) -> (-237.5, -49.5) projected
  line L60 (-237.5, -49.5) -> (-237.5, -60.5) projected
  line L61 (-237.5, -60.5) -> (-233.5, -60.5) projected
  line L62 (-233.5, -71.5) -> (-233.5, -60.5) projected
  line L63 (-233.5, -71.5) -> (-237.5, -71.5) projected
  line L64 (-237.5, -71.5) -> (-237.5, -82.5) projected
  line L65 (-237.5, -82.5) -> (-218.5, -82.5) projected
  line L66 (-218.5, -82.5) -> (-218.5, -78.5) projected
  line L67 (-199.5, -78.5) -> (-218.5, -78.5) projected
  line L68 (-199.5, -78.5) -> (-199.5, -82.5) projected
  line L69 (-199.5, -82.5) -> (-180.5, -82.5) projected
  line L70 (-180.5, -82.5) -> (-180.5, -78.5) projected
  line L71 (-161.5, -78.5) -> (-180.5, -78.5) projected
  line L72 (-161.5, -78.5) -> (-161.5, -82.5) projected
  line L73 (-161.5, -82.5) -> (-142.5, -82.5) projected
  line L74 (-142.5, -82.5) -> (-142.5, -78.5) projected
  line L75 (-123.5, -78.5) -> (-142.5, -78.5) projected
  line L76 (-123.5, -78.5) -> (-123.5, -82.5) projected
  line L77 (-123.5, -82.5) -> (-104.5, -82.5) projected
  line L78 (-104.5, -82.5) -> (-104.5, -78.5) projected
  line L79 (-85.5, -78.5) -> (-104.5, -78.5) projected
  line L80 (-85.5, -78.5) -> (-85.5, -82.5) projected
  line L81 (-85.5, -82.5) -> (-66.5, -82.5) projected
  line L82 (-66.5, -82.5) -> (-66.5, -78.5) projected
  line L83 (-47.5, -78.5) -> (-66.5, -78.5) projected
  line L84 (-47.5, -78.5) -> (-47.5, -82.5) projected
  line L85 (-47.5, -82.5) -> (-28.5, -82.5) projected
  line L86 (-28.5, -82.5) -> (-28.5, -78.5) projected
  line L87 (-9.5, -78.5) -> (-28.5, -78.5) projected
  line L88 (-9.5, -78.5) -> (-9.5, -82.5) projected
  line L89 (-9.5, -82.5) -> (9.5, -82.5) projected
  line L90 (9.5, -82.5) -> (9.5, -78.5) projected
  line L91 (28.5, -78.5) -> (9.5, -78.5) projected
  line L92 (28.5, -78.5) -> (28.5, -82.5) projected
  line L93 (28.5, -82.5) -> (47.5, -82.5) projected
  line L94 (47.5, -82.5) -> (47.5, -78.5) projected
  line L95 (66.5, -78.5) -> (47.5, -78.5) projected
  line L96 (66.5, -78.5) -> (66.5, -82.5) projected
  line L97 (66.5, -82.5) -> (85.5, -82.5) projected
  line L98 (85.5, -82.5) -> (85.5, -78.5) projected
  line L99 (104.5, -78.5) -> (85.5, -78.5) projected
  line L100 (104.5, -78.5) -> (104.5, -82.5) projected
  line L101 (104.5, -82.5) -> (123.5, -82.5) projected
  line L102 (123.5, -82.5) -> (123.5, -78.5) projected
  line L103 (142.5, -78.5) -> (123.5, -78.5) projected
  line L104 (142.5, -78.5) -> (142.5, -82.5) projected
  line L105 (142.5, -82.5) -> (161.5, -82.5) projected
  line L106 (161.5, -82.5) -> (161.5, -78.5) projected
  line L107 (180.5, -78.5) -> (161.5, -78.5) projected
  line L108 (180.5, -78.5) -> (180.5, -82.5) projected
  line L109 (180.5, -82.5) -> (199.5, -82.5) projected
  line L110 (199.5, -82.5) -> (199.5, -78.5) projected
  line L111 (218.5, -78.5) -> (199.5, -78.5) projected
  line L112 (-233.5, 66) -> (-226.5, 66) construction
  circle A7 centre (-226.5, 66) radius 1.65
  line L113 (-233.5, -71.5) -> (-233.5, -60.5) projected
  line L114 (-233.5, -66) -> (-226.5, -66) construction
  circle A8 centre (-226.5, -66) radius 1.65
  line L115 (-199.5, -78.5) -> (-218.5, -78.5) projected
  line L116 (-209, -78.5) -> (-209, -71.5) construction
  line L117 (-47.5, -78.5) -> (-66.5, -78.5) construction
  line L118 (-57, -78.5) -> (-57, -71.5) construction
  line L119 (218.5, -78.5) -> (199.5, -78.5) construction
  line L120 (209, -78.5) -> (209, -71.5) construction
  line L121 (233.5, -66) -> (226.5, -66) construction
  line L122 (233.5, 71.5) -> (233.5, 60.5) construction
  line L123 (233.5, 66) -> (226.5, 66) construction
  circle A9 centre (226.5, -66) radius 1.65
  circle A10 centre (209, -71.5) radius 1.65
  circle A11 centre (226.5, 66) radius 1.65
  circle A12 centre (-209, -71.5) radius 1.65
  circle A13 centre (-57, -71.5) radius 1.65
  point P0 (0, 0)
  dimension "d57" = 7
  dimension "d58" = 3.3
  dimension "d59" = 7
  dimension "d60" = 3.3
  dimension "d61" = 7
  dimension "d62" = 7
  dimension "d63" = 7
  dimension "d64" = 7
  dimension "d65" = 7
  dimension "d66" = 3.3
  dimension "d67" = 3.3
  dimension "d68" = 3.3
  dimension "d69" = 3.3
  dimension "d70" = 3.3
  constraints: 14 end point, 7 centre point, 7 coincident, 7 midpoint, 4 horizontal, 3 vertical
  measures "d57" distance of L112.start L112.end
  measures "d58" diameter of A7
  measures "d59" distance of L114.start L114.end
  measures "d60" diameter of A8
  measures "d61" distance of L116.start L116.end
  measures "d62" distance of L118.start L118.end
  measures "d63" distance of L120.start L120.end
  measures "d64" distance of L121.start L121.end
  measures "d65" distance of L123.start L123.end
  measures "d66" diameter of A9
  measures "d67" diameter of A10
  measures "d68" diameter of A11
  measures "d69" diameter of A12
  measures "d70" diameter of A13
extrude "Estrusione4" cut sketch "Schizzo5" against normal blind 10 contours A7 | A8 | A9 | A10 | A11 | A12 | A13
